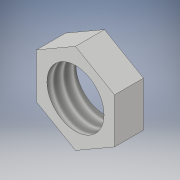
# Autodesk Inventor part: Nut
Saved by Autodesk Inventor 2019 (Build 230136000, 136)
## iProperties
Created: 2020-01-15
Part Number: Nut
Material: Generic
Document SubType Name: Modeling
Designer: 18186
Density: 1 g/cm^3
Appearance: Default
Author: 18186
Autodesk Inventor part; units mm, degrees
ref_plane "YZ Plane" through (0, 0, 0) normal (1, 0, 0) x (0, 1, 0)
ref_plane "XZ Plane" through (0, 0, 0) normal (0, 1, 0) x (-1, 0, 0)
ref_plane "XY Plane" through (0, 0, 0) normal (0, 0, 1) x (1, 0, 0)
sketch "Sketch1" plane through (0, 0, 0) normal (0, 0, 1) x (1, 0, 0)
  circle A0 centre (0, 0) radius 5
  line L0 (0, 7.8889) -> (6.832, 3.9445)
  line L1 (6.832, 3.9445) -> (6.832, -3.9445)
  line L2 (6.832, -3.9445) -> (0, -7.8889)
  line L3 (0, -7.8889) -> (-6.832, -3.9445)
  line L4 (-6.832, -3.9445) -> (-6.832, 3.9445)
  line L5 (-6.832, 3.9445) -> (0, 7.8889)
  dimension "d0" = 10
  constraints: 12 end point, 2 coincident, 1 centre point, 13 other
  measures "d0" diameter of A0
extrude "Extrusion1" add sketch "Sketch1" along normal blind 5.08
thread "Thread1" size "7/16-14 UNC" class "2B" standard "ANSI Unified Screw Threads" full length
body "Solid1"
